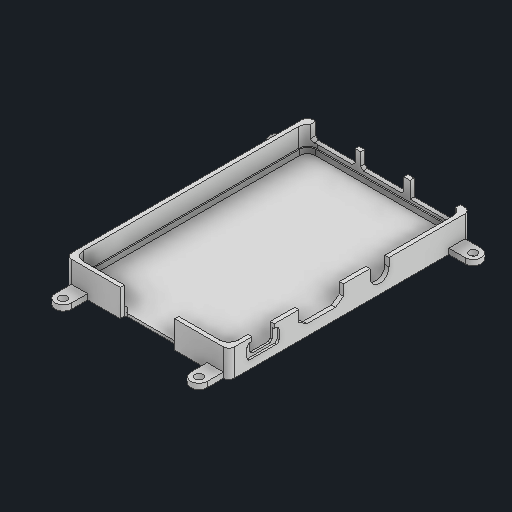
# Autodesk Inventor part: raspi_enclosure
Saved by Autodesk Inventor 2025 (Build 290162010, 162A)
## iProperties
Created: 2024-09-11
Part Number: raspi_enclosure
Material: Generic
Document SubType Name: Modeling
Designer: mihir
Density: 1 g/cm^3
Appearance: Default
Author: mihir
Autodesk Inventor part; units mm, degrees
ref_plane "YZ Plane" through (0, 0, 0) normal (1, 0, 0) x (0, 1, 0)
ref_plane "XZ Plane" through (0, 0, 0) normal (0, 1, 0) x (-1, 0, 0)
sketch "Sketch1" plane through (0, 0, 0) normal (0, 1, 0) x (-1, 0, 0)
  line L0 (2, 0) -> (58, 0)
  line L1 (60, -2) -> (60, -87)
  line L2 (58, -89) -> (2, -89)
  line L3 (0, -87) -> (0, -2)
  arc A0 (60, -2) -> (58, 0) centre (58, -2) ccw
  arc A1 (2, 0) -> (0, -2) centre (2, -2) ccw
  arc A2 (58, -89) -> (60, -87) centre (58, -87) ccw
  arc A3 (0, -87) -> (2, -89) centre (2, -87) ccw
  point P0 (0, 0)
  point P1 (60, 0)
  point P2 (0, -89)
  dimension "d0" = 89
  dimension "d1" = 60
  dimension "d2" = 2
  constraints: 8 end point, 8 point on circle, 8 tangent, 6 point on line, 4 centre point, 3 equal radius, 2 parallel, 1 horizontal, 1 perpendicular
  measures "d0" distance of point (0, -89) point (0, 0)
  measures "d1" distance of point (0, 0) point (60, 0)
  measures "d2" radius of A0
extrude "Extrusion1" add sketch "Sketch1" along normal blind 1
sketch "Sketch2" plane through (0, 1, 0) normal (0, 1, 0) x (1, 0, 0)
  line L0 (-60, 87) -> (-60, 2) projected
  line L1 (-58, 0) -> (-2, 0) projected
  line L2 (0, 2) -> (0, 87) projected
  line L3 (-2, 89) -> (-58, 89) projected
  line L4 (-2, 0) -> (-58, 0)
  line L5 (-60, 2) -> (-60, 87)
  line L6 (-58, 89) -> (-2, 89)
  line L7 (0, 87) -> (0, 2)
  arc A0 (-58, 89) -> (-60, 87) centre (-58, 87) ccw
  arc A1 (-60, 2) -> (-58, 0) centre (-58, 2) ccw
  arc A2 (-2, 0) -> (0, 2) centre (-2, 2) ccw
  arc A3 (0, 87) -> (-2, 89) centre (-2, 87) ccw
  line L8 (-55, 1.5) -> (-5, 1.5)
  line L9 (-1.5, 5) -> (-1.5, 84)
  line L10 (-5, 87.5) -> (-55, 87.5)
  line L11 (-58.5, 84) -> (-58.5, 5)
  arc A4 (-5, 1.5) -> (-1.5, 5) centre (-5, 5) ccw
  arc A5 (-58.5, 5) -> (-55, 1.5) centre (-55, 5) ccw
  arc A6 (-55, 87.5) -> (-58.5, 84) centre (-55, 84) ccw
  arc A7 (-1.5, 84) -> (-5, 87.5) centre (-5, 84) ccw
  point P0 (0, 0)
  point P1 (-60, 89)
  point P2 (-30, 89)
  point P3 (-2, 0)
  dimension "d5" = 2
  dimension "d6" = 1.5
  dimension "d7" = 1.5
  dimension "d8" = 1.5
  dimension "d9" = 1.5
  dimension "d10" = 3.5
  constraints: 16 end point, 16 point on circle, 16 tangent, 8 centre point, 6 equal radius, 5 point on line, 4 parallel, 2 horizontal, 2 perpendicular, 1 collinear, 1 midpoint
  measures "d5" radius of A0
  measures "d6" distance between parallel lines of L0 L11
  measures "d7" distance between parallel lines of L2 L9
  measures "d8" distance between parallel lines of L1 L8
  measures "d9" distance from line of point (-30, 89) L10
  measures "d10" radius of A4
extrude "Extrusion2" add sketch "Sketch2" along normal blind 9
sketch "Sketch4" plane through (0, 1, 0) normal (0, 1, 0) x (1, 0, 0)
  line L0 (-55, 1.5) -> (-5, 1.5)
  line L1 (-1.5, 5) -> (-1.5, 84)
  line L2 (-5, 87.5) -> (-55, 87.5)
  line L3 (-58.5, 84) -> (-58.5, 5)
  line L4 (-58.5, 5) -> (-58.5, 84) projected
  line L5 (-5, 1.5) -> (-55, 1.5) projected
  line L6 (-1.5, 84) -> (-1.5, 5) projected
  line L7 (-55, 87.5) -> (-5, 87.5) projected
  arc A0 (-55, 87.5) -> (-58.5, 84) centre (-55, 84) ccw
  arc A1 (-58.5, 5) -> (-55, 1.5) centre (-55, 5) ccw
  arc A2 (-5, 1.5) -> (-1.5, 5) centre (-5, 5) ccw
  arc A3 (-1.5, 84) -> (-5, 87.5) centre (-5, 84) ccw
  line L8 (-55, 2) -> (-5, 2)
  line L9 (-2, 5) -> (-2, 84)
  line L10 (-5, 87) -> (-55, 87)
  line L11 (-58, 84) -> (-58, 5)
  arc A4 (-58, 5) -> (-55, 2) centre (-55, 5) ccw
  arc A5 (-5, 2) -> (-2, 5) centre (-5, 5) ccw
  arc A6 (-2, 84) -> (-5, 87) centre (-5, 84) ccw
  arc A7 (-55, 87) -> (-58, 84) centre (-55, 84) ccw
  point P0 (0, 0)
  dimension "d13" = 3.5
  dimension "d14" = 0.5
  dimension "d15" = 0.5
  dimension "d16" = 0.5
  dimension "d17" = 0.5
  dimension "d18" = 3
  dimension "d19" = 3
  constraints: 16 end point, 16 point on circle, 16 tangent, 8 centre point, 5 equal radius, 4 collinear, 4 parallel, 2 horizontal, 2 perpendicular
  measures "d13" radius of A0
  measures "d14" distance between parallel lines of L4 L11
  measures "d15" distance between parallel lines of L1 L9
  measures "d16" distance between parallel lines of L0 L8
  measures "d17" distance between parallel lines of L2 L10
  measures "d18" radius of A4
  measures "d19" radius of A5
extrude "Extrusion3" add sketch "Sketch4" along normal blind 2
sketch "Sketch5" plane through (0, 10, 0) normal (0, 1, 0) x (1, 0, 0)
  line L0 (-40, 0) -> (-20, 0)
  line L1 (-20, 0) -> (-20, 1.5)
  line L2 (-20.5, 2) -> (-39.5, 2)
  line L3 (-40, 1.5) -> (-40, 0)
  arc A0 (-39.5, 2) -> (-40, 1.5) centre (-39.5, 1.5) ccw
  arc A1 (-20, 1.5) -> (-20.5, 2) centre (-20.5, 1.5) ccw
  line L4 (-30, 0) -> (-30, 2) construction
  line L5 (-58, 0) -> (-2, 0) construction
  line L6 (-30, 0) -> (-30, 1.5) construction
  line L7 (-5, 1.5) -> (-55, 1.5) construction
  line L8 (-58, 0) -> (-2, 0) construction
  point P0 (0, 0)
  point P1 (-40, 2)
  dimension "d22" = 2
  dimension "d23" = 20
  dimension "d24" = 0.5
  constraints: 12 end point, 4 midpoint, 4 point on circle, 4 tangent, 2 centre point, 2 collinear, 2 parallel, 2 point on line, 1 equal radius, 1 horizontal, 1 perpendicular
  measures "d22" distance of point (-40, 2) L0.start
  measures "d23" distance of L0.start L0.end
  measures "d24" radius of A0
extrude "Extrusion4" cut sketch "Sketch5" against normal up to surface (10 mm away)
sketch "Sketch6" plane through (0, 0, -2) normal (1, 0, 0) x (0, 0, -1)
  line L0 (23.75, 10) -> (40.25, 10)
  line L1 (40.25, 10) -> (40.25, 6)
  line L2 (3, 3) -> (82, 3) projected
  line L3 (23.75, 10) -> (23.75, 6)
  line L4 (23.75, 6) -> (26.75, 4)
  line L5 (26.75, 4) -> (37.25, 4)
  line L6 (37.25, 4) -> (40.25, 6)
  line L7 (32, 10) -> (32, 4) construction
  line L8 (0, 10) -> (85, 10) construction
  line L9 (-2, 0) -> (-2, 10) construction
  dimension "d27" = 16.5
  dimension "d28" = 4
  dimension "d29" = 10.5
  dimension "d30" = 6
  dimension "d31" = 25.75
  constraints: 14 end point, 2 equal length, 2 midpoint, 2 perpendicular, 1 collinear, 1 horizontal, 1 vertical
  measures "d27" distance of L0.start L0.end
  measures "d28" distance of L0.end L1.end
  measures "d29" distance of L4.end L5.end
  measures "d30" distance of L7.start L7.end
  measures "d31" distance between parallel lines of L9 L3
extrude "Extrusion5" cut sketch "Sketch6" against normal up to surface (1.5 mm away)
sketch "Sketch7" plane through (0, 0, -2) normal (1, 0, 0) x (0, 0, -1)
  line L0 (50, 10) -> (57, 10)
  line L1 (57, 10) -> (57, 7)
  line L2 (57, 7) -> (50, 7)
  line L3 (50, 7) -> (50, 10)
  line L4 (40.25, 10) -> (85, 10) projected
  arc A0 (50, 7) -> (57, 7) centre (53.5, 7) ccw
  line L5 (40.25, 10) -> (40.25, 6) projected
  point P0 (-2, 0)
  dimension "d34" = 7
  dimension "d35" = 3
  dimension "d36" = 9.75
  constraints: 8 end point, 2 parallel, 2 point on circle, 1 centre point, 1 collinear, 1 horizontal, 1 midpoint, 1 perpendicular
  measures "d34" distance of L0.start L0.end
  measures "d35" distance of L2.end L0.start
  measures "d36" distance between parallel lines of L5 L3
extrude "Extrusion6" cut sketch "Sketch7" against normal up to surface (1.5 mm away)
sketch "Sketch8" plane through (0, 0, -2) normal (1, 0, 0) x (0, 0, -1)
  line L0 (6.5, 10) -> (14.7, 10)
  line L1 (14.7, 10) -> (14.7, 4.8)
  line L2 (14.7, 4.8) -> (6.5, 4.8)
  line L3 (6.5, 4.8) -> (6.5, 10)
  line L4 (6.5, 4.8) -> (7.3, 4)
  line L5 (7.3, 4) -> (13.9, 4)
  line L6 (13.9, 4) -> (14.7, 4.8)
  line L7 (0, 10) -> (23.75, 10) projected
  line L8 (23.75, 6) -> (23.75, 10) projected
  point P0 (-2, 0)
  point P1 (10.6, 4)
  dimension "d39" = 8.2
  dimension "d40" = 5.2
  dimension "d41" = 6.6
  dimension "d42" = 6
  dimension "d43" = 9.05
  constraints: 14 end point, 2 horizontal, 2 parallel, 2 perpendicular, 1 collinear, 1 midpoint
  measures "d39" distance of L0.start L0.end
  measures "d40" distance of L2.end L0.start
  measures "d41" distance of L4.end L5.end
  measures "d42" distance from line of point (10.6, 4) L0
  measures "d43" distance between parallel lines of L8 L1
extrude "Extrusion7" cut sketch "Sketch8" against normal up to surface (1.5 mm away)
sketch "Sketch9" plane through (0, 0, -2) normal (1, 0, 0) x (0, 0, -1)
  line L0 (5.6855, 8.466) -> (15.5145, 8.466)
  line L1 (16.5145, 7.466) -> (16.5145, 4.078)
  line L2 (15.5145, 3.078) -> (5.6855, 3.078)
  line L3 (4.6855, 4.078) -> (4.6855, 7.466)
  arc A0 (5.6855, 8.466) -> (4.6855, 7.466) centre (5.6855, 7.466) ccw
  arc A1 (4.6855, 4.078) -> (5.6855, 3.078) centre (5.6855, 4.078) ccw
  arc A2 (15.5145, 3.078) -> (16.5145, 4.078) centre (15.5145, 4.078) ccw
  arc A3 (16.5145, 7.466) -> (15.5145, 8.466) centre (15.5145, 7.466) ccw
  line L4 (13.9, 4) -> (7.3, 4) projected
  line L5 (16.5145, 5.772) -> (14.7, 5.772) construction
  line L6 (14.7, 4.8) -> (14.7, 10) construction
  line L7 (4.6855, 5.772) -> (6.5, 5.772) construction
  line L8 (6.5, 10) -> (6.5, 4.8) construction
  point P0 (-2, 0)
  dimension "d46" = 5.388
  dimension "d47" = 11.829
  dimension "d48" = 1
  dimension "d49" = 0.922
  constraints: 12 end point, 8 point on circle, 8 tangent, 4 centre point, 3 equal radius, 3 point on line, 2 horizontal, 2 midpoint, 2 parallel, 1 collinear, 1 perpendicular
  measures "d46" distance between parallel lines of L2 L0
  measures "d47" distance between parallel lines of L1 L3
  measures "d48" radius of A0
  measures "d49" distance between parallel lines of L4 L2
extrude "Extrusion8" cut sketch "Sketch9" against normal blind 0.75
sketch "Sketch10" plane through (-2, 0, -89) normal (0, 0, -1) x (-1, 0, 0)
  line L0 (1.75, 10) -> (18.75, 10)
  line L1 (18.75, 10) -> (18.75, 4)
  line L2 (18.75, 4) -> (1.75, 4)
  line L3 (1.75, 4) -> (1.75, 10)
  line L4 (0, 10) -> (56, 10) projected
  line L5 (-2, 0) -> (-2, 10) projected
  dimension "d52" = 17
  dimension "d53" = 6
  dimension "d54" = 3.75
  constraints: 8 end point, 2 parallel, 1 collinear, 1 horizontal, 1 perpendicular
  measures "d52" distance of L0.start L0.end
  measures "d53" distance of L2.end L0.start
  measures "d54" distance between parallel lines of L5 L3
extrude "Extrusion9" cut sketch "Sketch10" against normal blind 2
sketch "Sketch11" plane through (-2, 0, -89) normal (0, 0, -1) x (-1, 0, 0)
  line L0 (21, 10) -> (37, 10)
  line L1 (37, 10) -> (37, 5.4)
  line L2 (37, 5.4) -> (36, 4.4)
  line L3 (36, 4.4) -> (22, 4.4)
  line L4 (22, 4.4) -> (21, 5.4)
  line L5 (21, 5.4) -> (21, 10)
  line L6 (29, 10) -> (29, 4.4) construction
  line L7 (18.75, 10) -> (56, 10) construction
  line L8 (18.75, 10) -> (18.75, 4) construction
  line L9 (55, 10) -> (55, 5.4)
  line L10 (39, 10) -> (55, 10)
  line L11 (39, 5.4) -> (39, 10)
  line L12 (40, 4.4) -> (39, 5.4)
  line L13 (54, 4.4) -> (40, 4.4)
  line L14 (55, 5.4) -> (54, 4.4)
  line L15 (37, 20) -> (37, 15.4)
  line L16 (21, 20) -> (37, 20)
  line L17 (21, 15.4) -> (21, 20)
  line L18 (22, 14.4) -> (21, 15.4)
  line L19 (36, 14.4) -> (22, 14.4)
  line L20 (37, 15.4) -> (36, 14.4)
  line L21 (55, 20) -> (55, 15.4)
  line L22 (39, 20) -> (55, 20)
  line L23 (39, 15.4) -> (39, 20)
  line L24 (40, 14.4) -> (39, 15.4)
  line L25 (54, 14.4) -> (40, 14.4)
  line L26 (55, 15.4) -> (54, 14.4)
  point P0 (-2, 0)
  point P1 (47, 10)
  point P2 (47, 4.4)
  point P3 (29, 20)
  point P4 (29, 14.4)
  point P5 (47, 20)
  point P6 (47, 14.4)
  dimension "d57" = 16
  dimension "d58" = 14
  dimension "d59" = 4.6
  dimension "d60" = 5.6
  dimension "d61" = 2.25
  dimension "d64" = 18
  dimension "d67" = 10
  constraints: 50 end point, 3 collinear, 3 parallel, 2 horizontal, 2 midpoint, 2 vertical, 1 perpendicular, 40 other
  measures "d57" distance of L0.start L0.end
  measures "d58" distance of L2.end L3.end
  measures "d59" distance of L4.end L0.start
  measures "d60" distance of L6.start L6.end
  measures "d61" distance between parallel lines of L8 L5
  measures "d64" distance of L0.end L9.start
  measures "d67" distance of L0.end L15.start
extrude "Extrusion10" cut sketch "Sketch11" against normal blind 2 contours L0 L1 L2 L3 L4 L5 | L9 L14 L13 L12 L11 L10
sketch "Sketch12" plane through (0, 0, 0) normal (0, -1, 0) x (1, 0, 0)
  arc A0 (0, -2) -> (-2, 0) centre (-2, -2) ccw projected
  line L0 (-2, 0) -> (-8, 0)
  line L1 (-8, 0) -> (-8, 6)
  line L2 (-8, 6) -> (-2, 6)
  line L3 (-2, 6) -> (-2, 0)
  circle A1 centre (-5, 6) radius 3
  circle A2 centre (-5, 6) radius 1.5
  arc A3 (-2, -89) -> (0, -87) centre (-2, -87) ccw projected
  line L4 (0, -87) -> (6, -87)
  line L5 (6, -87) -> (6, -81)
  line L6 (6, -81) -> (0, -81)
  line L7 (0, -81) -> (0, -87)
  circle A4 centre (6, -84) radius 3
  circle A5 centre (6, -84) radius 1.5
  point P0 (0, 0)
  dimension "d72" = 6
  dimension "d75" = 6
  dimension "d73" = 6
  dimension "d74" = 3
  dimension "d76" = 6
  dimension "d77" = 3
  constraints: 16 end point, 4 parallel, 2 centre point, 2 coincident, 2 horizontal, 2 midpoint, 2 perpendicular, 6 other
  measures "d73" distance of L0.end L1.end
  measures "d74" diameter of A2
  measures "d76" distance of L5.end L6.end
  measures "d77" diameter of A5
extrude "Extrusion11" add sketch "Sketch12" against normal blind 2 contours L0 L1 A1 L3 | A1 L2 A2 | L2 A2 A1 | L7 L6 A4 L4 | A4 L5 A5 | L5 A5 A4
ref_plane "Work Plane1" through (-30, 0, -2) normal (1, 0, 0) x (0, 0, -1)
mirror "Mirror1" about plane through (-30, 0, -2) normal (1, 0, 0) of "Extrusion11"
body "Solid1"
